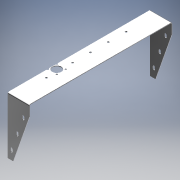
# Autodesk Inventor part: Turret Support Brace
Saved by Autodesk Inventor 2019.4 (Build 234330000, 330)
## iProperties
Created: 2020-01-12
Part Number: Turret Support Brace
Material: Aluminum 6061
Document SubType Name: Sheet Metal
Designer: admin
Density: 2.7 g/cm^3
Sheet Metal Rule: Default_mm
Appearance: Aluminum - Flat
Mass: 291.389 g
Surface Area: 772.551 cm^2
Volume: 107.922 cm^3
Author: admin
Autodesk Inventor part; units mm, degrees
ref_plane "YZ Plane" through (0, 0, 0) normal (1, 0, 0) x (0, 1, 0)
ref_plane "XZ Plane" through (0, 0, 0) normal (0, 1, 0) x (-1, 0, 0)
ref_plane "XY Plane" through (0, 0, 0) normal (0, 0, 1) x (1, 0, 0)
sketch "Sketch1" plane through (0, 0, 0) normal (0, 1, 0) x (-1, 0, 0)
  line L0 (-30, 200) -> (30, 200)
  line L1 (30, 200) -> (30, -200)
  line L2 (30, -200) -> (-30, -200)
  line L3 (-30, -200) -> (-30, 200)
  line L4 (-30, 200) -> (30, -200) construction
  line L5 (30, 200) -> (-30, -200) construction
  point P0 (0, 0)
  dimension "d0" = 60
  dimension "d1" = 400
  measures "d0" distance of L1.end L2.end
  measures "d1" distance of L0.end L1.end
extrude "Plate1" add sketch "Sketch1" along normal blind 2
sketch "Sketch2" plane through (-30, 2, 198) normal (0, 0, 1) x (1, 0, 0)
  line L0 (60, 0) -> (0, 0)
  line L1 (0, 0) -> (0, -160)
  line L2 (0, -160) -> (60, -160)
  line L3 (60, -160) -> (60, 0)
  constraints: 6 end point, 1 horizontal, 1 perpendicular, 1 vertical
edge flange "Flange1" height 160 angle 90 thickness 2 bend radius 2 thickness toward (0, 0, 1) relief tear relief width 2 relief depth 1 corner gap 2 corner form 0 edges at (0, 0, 200) (0, 0, -200) wall of the first edge with corners at (30, 2, 198) (-30, 2, 198) (-30, -158, 198) (30, -158, 198)
bend "Bend1"
corner "Corner1"
sketch "Sketch3" plane through (0, 2, 0) normal (0, 1, 0) x (1, 0, 0)
  circle A0 centre (-10.5, -111.5239) radius 2.75 projected
  circle A1 centre (-10.5, -38.4761) radius 2.75 projected
  circle A2 centre (-4.3429, -88.5614) radius 2.25 projected
  circle A3 centre (-4.3429, -63.8126) radius 2.25 projected
  circle A4 centre (-29.0916, -88.5614) radius 2.25 projected
  circle A5 centre (-29.0916, -63.8126) radius 2.25 projected
  circle A6 centre (-10.5, 11.5239) radius 2.75 projected
  circle A7 centre (-10.5, 61.5239) radius 2.75 projected
  circle A8 centre (-10.5, 111.5239) radius 2.75 projected
  circle A9 centre (-16.7173, -76.187) radius 12.75 projected
  point P0 (0, 0)
extrude "Extrusion1" cut sketch "Sketch3" against normal through all
fillet "Fillet1" radius 3 4 edges at (-30, 1, 90.6199) (-30, 1, 86.5029) (-30, 1, 65.8711) (-30, 1, 61.7541)
sketch "Sketch4" plane through (-30, -158, 200) normal (0, 0, 1) x (1, 0, 0)
  line L0 (0, 0) -> (60, 0) projected
  line L1 (15, 0) -> (60, 128.9325)
  line L2 (60, 156) -> (60, 0) projected
  line L3 (10.486, 25) -> (43.4386, 119.4147) construction
  circle A0 centre (43.4386, 119.4147) radius 2.75 construction
  circle A1 centre (10.486, 25) radius 2.75 construction
  circle A2 centre (26.9623, 72.2073) radius 2.75 construction
  line L4 (43.4386, 116.4147) -> (43.4386, 122.4147) construction
  line L5 (46.1886, 116.4147) -> (46.1886, 122.4147)
  line L6 (40.6886, 122.4147) -> (40.6886, 116.4147)
  arc A3 (40.6886, 116.4147) -> (46.1886, 116.4147) centre (43.4386, 116.4147) ccw
  arc A4 (46.1886, 122.4147) -> (40.6886, 122.4147) centre (43.4386, 122.4147) ccw
  line L7 (26.9623, 69.2073) -> (26.9623, 75.2073) construction
  line L8 (29.7123, 69.2073) -> (29.7123, 75.2073)
  line L9 (24.2123, 75.2073) -> (24.2123, 69.2073)
  arc A5 (24.2123, 69.2073) -> (29.7123, 69.2073) centre (26.9623, 69.2073) ccw
  arc A6 (29.7123, 75.2073) -> (24.2123, 75.2073) centre (26.9623, 75.2073) ccw
  line L10 (10.486, 22) -> (10.486, 28) construction
  line L11 (13.236, 22) -> (13.236, 28)
  line L12 (7.736, 28) -> (7.736, 22)
  arc A7 (7.736, 22) -> (13.236, 22) centre (10.486, 22) ccw
  arc A8 (13.236, 28) -> (7.736, 28) centre (10.486, 28) ccw
  point P0 (30, 158)
  dimension "d17" = 45
  dimension "d20" = 70.76
  dimension "d21" = 5.5
  dimension "d22" = 5.5
  dimension "d23" = 5.5
  dimension "d24" = 100
  dimension "d25" = 25
  dimension "d26" = 12.5
  dimension "d27" = 3
  dimension "d28" = 5.5
  dimension "d29" = 3
  dimension "d30" = 5.5
  dimension "d31" = 3
  dimension "d32" = 5.5
  constraints: 28 end point, 12 point on circle, 12 tangent, 9 centre point, 5 parallel, 4 midpoint, 2 coincident, 2 point on line, 2 vertical
  measures "d17" distance from line of L2 L1.start
  measures "d20" angle of L0 L1
  measures "d21" diameter of A0
  measures "d22" diameter of A1
  measures "d23" diameter of A2
  measures "d24" distance between centres of A1 A0
  measures "d25" distance from line of L0 L3.start
  measures "d26" distance between parallel lines of L1 L3
  measures "d27" distance of A0.centre L4.end
  measures "d28" diameter of A4
  measures "d29" distance of A2.centre L7.end
  measures "d30" diameter of A6
  measures "d31" distance of A1.centre L10.end
  measures "d32" diameter of A8
extrude "Extrusion2" cut sketch "Sketch4" against normal through all
equation "\"d2\" = Thickness"
equation "\"d3\" = BendReliefWidth"
equation "\"d4\" = BendReliefDepth"
equation "\"d5\" = MinimumRemnant"
equation "\"d6\" = TransitionRadius"
equation "\"d9\" = BendRadius"
equation "\"d10\" = CornerReliefSize"
equation "\"d11\" = GapSize"
equation "\"d12\" = JacobiRadiusSize"
equation "\"BendRadius\" = Thickness"
equation "\"BendReliefWidth\" = Thickness"
equation "\"BendReliefDepth\" = 0.5 * Thickness"
equation "\"CornerReliefSize\" = 4 * Thickness"
equation "\"MinimumRemnant\" = 2 * Thickness"
equation "\"TransitionRadius\" = BendRadius"
equation "\"JacobiRadiusSize\" = BendRadius"
equation "\"GapSize\" = Thickness"
equation "\"Thickness\" = 2"
body "Solid1"
